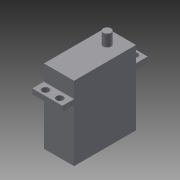
# Autodesk Inventor part: SimplifiedServo
Saved by Autodesk Inventor 2014 (Build 180170000, 170)
## iProperties
Created: 2013-09-08
Part Number: SimplifiedServo
Material: Generic
Document SubType Name: Modeling
Designer: Medrimonia
Density: 1 g/cm^3
Appearance: Default
ServoCoreWidth: 11.400 mm
ServoSpacing: 0.200 mm
ServoCoreLength: 23.500 mm
ServoFixationLength: 4.400 mm
ServoCoreToFixation: 2.400 mm
ServoEdgeToFixation: 3,000 mm
ServoScrewDiameter: 2,000 mm
ServoScrewDiameterRequired: 2,600 mm
ServoHeadScrewTrace: 4,500 mm
ServoHeadScrewThickness: 2,500 mm
ServoExtendedSpacing: 1,000 mm
ServoAxisToCenter: 6,500 mm
Author: Medrimonia
Autodesk Inventor part; units mm, degrees
ref_plane "YZ Plane" through (0, 0, 0) normal (1, 0, 0) x (0, 1, 0)
ref_plane "XZ Plane" through (0, 0, 0) normal (0, 1, 0) x (-1, 0, 0)
ref_plane "XY Plane" through (0, 0, 0) normal (0, 0, 1) x (1, 0, 0)
sketch "Sketch1" plane through (0, 0, 0) normal (0, 0, 1) x (1, 0, 0)
  line L0 (-5.7, -11.75) -> (5.7, -11.75)
  line L1 (5.7, -11.75) -> (5.7, 11.75)
  line L2 (5.7, 11.75) -> (-5.7, 11.75)
  line L3 (-5.7, 11.75) -> (-5.7, -11.75)
  line L4 (-5.7, -11.75) -> (5.7, 11.75) construction
  line L5 (5.7, -11.75) -> (-5.7, 11.75) construction
  line L6 (5.7, 11.75) -> (-5.7, 11.75)
  line L7 (-5.7, 11.75) -> (-5.7, 16.15)
  line L8 (-5.7, 16.15) -> (5.7, 16.15)
  line L9 (5.7, 16.15) -> (5.7, 11.75)
  circle A0 centre (-2.7, 14.15) radius 1.3
  circle A1 centre (2.7, 14.15) radius 1.3
  circle A2 centre (-2.7, -14.15) radius 1.3
  circle A3 centre (2.7, -14.15) radius 1.3
  line L10 (-5.7, -11.75) -> (5.7, -11.75)
  line L11 (5.7, -11.75) -> (5.7, -16.15)
  line L12 (5.7, -16.15) -> (-5.7, -16.15)
  line L13 (-5.7, -16.15) -> (-5.7, -11.75)
  point P0 (0, 0)
  dimension "d0" = 11.4
  dimension "d1" = 23.5
  dimension "d2" = 4.4
  dimension "d3" = 2.6
  dimension "d4" = 3
  dimension "d5" = 2.4
  dimension "d6" = 4.4
  dimension "d7" = 3
  dimension "d8" = 3
  dimension "d9" = 3
  dimension "d10" = 2.4
  dimension "d11" = 2.4
  dimension "d18" = 2.4
  constraints: 28 end point, 8 parallel, 4 centre point, 3 equal radius, 3 horizontal, 3 perpendicular, 2 midpoint
  measures "d0" distance of L2.end L1.end
  measures "d1" distance of L1.end L0.end
  measures "d2" distance of L6.end L7.end
  measures "d3" diameter of A0
  measures "d4" distance from line of L7 A0.centre
  measures "d5" distance from line of L2 A0.centre
  measures "d6" distance of L10.end L11.end
  measures "d7" distance from line of L9 A1.centre
  measures "d8" distance from line of L11 A3.centre
  measures "d9" distance from line of L13 A2.centre
  measures "d10" distance from line of L0 A2.centre
  measures "d11" distance from line of L0 A3.centre
  measures "d18" distance from line of A1.centre L2
extrude "Extrusion1" add sketch "Sketch1" along normal blind 8 and the other way blind 20 contours L3 L2 L1 L0
extrude "Extrusion2" add sketch "Sketch1" along normal blind 2 contours L7 L8 L9 L2
extrude "Extrusion3" add sketch "Sketch1" along normal blind 2 contours L0 L11 L12 L13
sketch "Sketch2" plane through (0, 0, 8) normal (0, 0, 1) x (1, 0, 0)
  line L0 (5.7, -11.75) -> (5.7, 11.75) projected
  circle A0 centre (-0.015, 6.5) radius 1.5
  point P0 (0, 0)
  dimension "d37" = 3
  dimension "d38" = 5.715
  dimension "d39" = 6.5
  constraints: 1 centre point
  measures "d37" diameter of A0
  measures "d38" distance from line of L0 A0.centre
  measures "d39" distance of point (0, 0) A0.centre
extrude "Extrusion4" add sketch "Sketch2" along normal blind 4.5
equation "\"d0\" = ServoCoreWidth"
equation "\"d1\" = ServoCoreLength"
equation "\"d2\" = ServoFixationLength"
equation "\"d4\" = ServoEdgeToFixation"
equation "\"d5\" = ServoCoreToFixation"
equation "\"d6\" = ServoFixationLength"
equation "\"d7\" = ServoEdgeToFixation"
equation "\"d8\" = ServoEdgeToFixation"
equation "\"d9\" = ServoEdgeToFixation"
equation "\"d10\" = ServoCoreToFixation"
equation "\"d11\" = ServoCoreToFixation"
equation "\"d18\" = ServoCoreToFixation"
equation "\"d39\" = ServoAxisToCenter"
equation "\"ServoCoreToFixation\" = 2.4"
equation "\"ServoEdgeToFixation\" = 3"
equation "\"ServoCoreWidth\" = 11.4"
equation "\"ServoSpacing\" = 0.2"
equation "\"ServoCoreLength\" = 23.5"
equation "\"ServoFixationLength\" = 4.4"
equation "\"ServoScrewDiameter\" = 2"
equation "\"ServoHeadScrewTrace\" = 4.5"
equation "\"ServoHeadScrewThickness\" = 2.5"
equation "\"ServoExtendedSpacing\" = 1"
equation "\"ServoAxisToCenter\" = 6.5"
body "Solid1"
